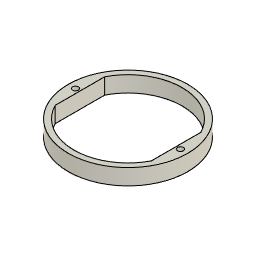
Electrical Box Spacers (Autodesk Fusion 360 design; units mm, degrees)
Autodesk Fusion 360 part; units mm, degrees
sketch "Base" plane through (0, 0, 0) normal (0, 0, 1) x (1, 0, 0) in component "Spacer (9mm)"
  circle A0 centre (0, 0) radius 33.85
  circle A1 centre (0, 0) radius 30.65
  circle A2 centre (-29.75, 0) radius 1.65
  circle A3 centre (29.75, 0) radius 1.65
  line L0 (-27.25, 14.0307) -> (-27.25, -14.0307)
  line L1 (27.25, 14.0307) -> (27.25, -14.0307)
  dimension "d1" = 67.7
  dimension "d2" = 61.3
  dimension "d3" = 3.3
  dimension "d4" = 29.75
  dimension "d5" = 3.3
  dimension "d6" = 29.75
  dimension "d7" = 27.25
  dimension "d8" = 27.25
  constraint coincident A0.centre A1.centre
  constraint concentric A0 A1
  constraint coincident A1 L0.start
  constraint coincident A1 L0.end
  constraint vertical L0
  constraint coincident A1 L1.start
  constraint coincident A1 L1.end
  constraint vertical L1
  measures "d1" diameter of A0
  measures "d2" diameter of A1
  measures "d3" diameter of A2
  measures "d4" distance of A0.centre A2.centre
  measures "d5" diameter of A3
  measures "d6" distance of A0.centre A3.centre
  measures "d7" distance of A0.centre L0
  measures "d8" distance of A0.centre L1
extrude "Extrude1" add sketch "Base" along normal blind 9 contours A0 | A1 A3 L1 | A1 A2 L0 in component "Spacer (9mm)"
component "Electrical Box Spacers" placed x (1, 0, 0) y (0, 1, 0) z (0, 0, 1) at (0, 0, 0)
component "Spacer (9mm)" placed x (1, 0, 0) y (0, 1, 0) z (0, 0, 1) at (0, 0, 0) in component "Electrical Box Spacers"
named bodies: "Spacer (9mm)"
